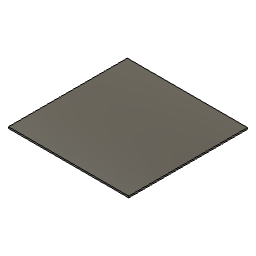
_MDF walls.563d6392-8aeb-4b5f-a8dd-61cc84657718 (Autodesk Fusion 360 design; units mm, degrees)
Autodesk Fusion 360 part; units mm, degrees
sketch "Sketch1" plane through (0, 0, 0) normal (0, 0, 1) x (1, 0, 0)
  line L0 (0, 0) -> (500, 0)
  line L1 (500, 0) -> (500, 494)
  line L2 (500, 494) -> (0, 494)
  line L3 (0, 494) -> (0, 0)
  dimension "d1" = 500
  dimension "d2" = 494
  constraint horizontal L0
  constraint vertical L1
  constraint horizontal L2
  constraint vertical L3
  constraint coincident L0.start L3.end
  measures "d1" distance of L0.start L0.end
  measures "d2" distance of L0.start L2.end
extrude "Extrude1" add sketch "Sketch1" along normal blind 6
